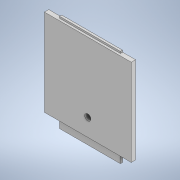
# Autodesk Inventor part: body_right
Saved by Autodesk Inventor 2022 (Build 260153000, 153)
## iProperties
Created: 2022-10-16
Part Number: body_right
Material: 一般
Document SubType Name: Modeling
Designer: haya
Density: 1 g/cm^3
Appearance: 既定
Author: haya
Autodesk Inventor part; units mm, degrees
ref_plane "YZ Plane" through (0, 0, 0) normal (1, 0, 0) x (0, 1, 0)
ref_plane "XZ Plane" through (0, 0, 0) normal (0, 1, 0) x (-1, 0, 0)
ref_plane "XY Plane" through (0, 0, 0) normal (0, 0, 1) x (1, 0, 0)
sketch "スケッチ1" plane through (0, 0, 0) normal (0, 0, 1) x (1, 0, 0)
  line L0 (0, 0) -> (100, 0)
  line L1 (100, 0) -> (100, 100)
  line L2 (100, 100) -> (0, 100)
  line L3 (0, 100) -> (0, 0)
  dimension "d0" = 100
  dimension "d1" = 100
  constraints: 8 end point, 2 parallel, 1 horizontal, 1 perpendicular
  measures "d0" distance of L0.start L0.end
  measures "d1" distance of L2.end L0.start
extrude "押し出し1" add sketch "スケッチ1" along normal blind 5
sketch "スケッチ2" plane through (0, 0, 0) normal (0, -1, 0) x (1, 0, 0)
  line L0 (100, 5) -> (0, 5) projected
  line L1 (50, 5) -> (50, 0) construction
  line L2 (100, 0) -> (0, 0) projected
  line L3 (85, 0) -> (15, 0)
  line L4 (15, 0) -> (15, 2.5)
  line L5 (15, 2.5) -> (85, 2.5)
  line L6 (85, 2.5) -> (85, 0)
  point P0 (15, 0)
  dimension "d4" = 70
  dimension "d5" = 2.5
  constraints: 10 end point, 2 midpoint, 2 parallel, 1 horizontal, 1 perpendicular, 1 point on line, 1 other
  measures "d4" distance of L4.end L5.end
  measures "d5" distance between parallel lines of L2 L5
extrude "押し出し2" add sketch "スケッチ2" along normal blind 10
sketch "スケッチ3" plane through (0, 0, 5) normal (0, 0, 1) x (1, 0, 0)
  line L0 (100, 100) -> (0, 100) projected
  line L1 (50, 100) -> (50, 0) construction
  line L2 (15, 0) -> (85, 0) projected
  point P0 (0, 0)
  point P1 (50, 20)
  dimension "d15" = 20
  constraints: 2 end point, 2 midpoint, 1 point on line
  measures "d15" distance from line of point (50, 20) L2
hole "穴1" at (50, 20, 5) direction (0, 0, -1) diameter 7 end through all
sketch "スケッチ5" plane through (0, 100, 0) normal (0, 1, 0) x (1, 0, 0)
  line L0 (53.5, -5) -> (46.5, -5) projected
  line L1 (50, -5) -> (50, 0) construction
  line L2 (46.5, 0) -> (53.5, 0) projected
  line L3 (100, 0) -> (0, 0) projected
  line L4 (15, 0) -> (85, 0)
  line L5 (85, 0) -> (85, -2.5)
  line L6 (85, -2.5) -> (15, -2.5)
  line L7 (15, -2.5) -> (15, 0)
  dimension "d25" = 2.5
  dimension "d26" = 70
  constraints: 10 end point, 2 midpoint, 2 parallel, 1 horizontal, 1 perpendicular, 1 point on line, 1 other
  measures "d25" distance between parallel lines of L6 L3
  measures "d26" distance of L5.end L6.end
extrude "押し出し3" add sketch "スケッチ5" along normal blind 2
